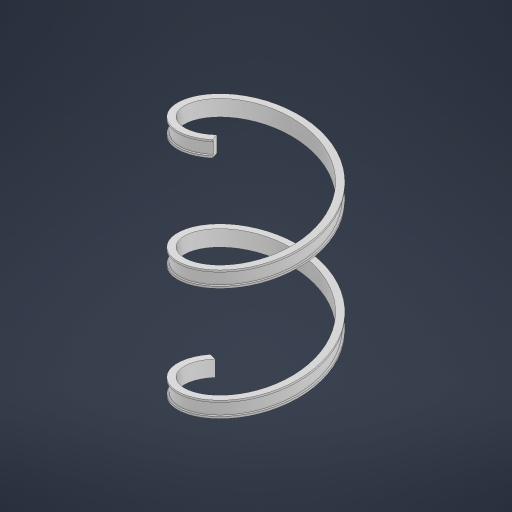
# Autodesk Inventor part: standalone
Saved by Autodesk Inventor 2023 (Build 270158000, 158)
## iProperties
Created: 2022-06-25
Part Number: standalone
Material: Generic
Document SubType Name: Modeling
Designer: bananenbrot
Density: 1 g/cm^3
Appearance: Default
Author: bananenbrot
Autodesk Inventor part; units mm, degrees
ref_plane "YZ Plane" through (0, 0, 0) normal (1, 0, 0) x (0, 1, 0)
ref_plane "XZ Plane" through (0, 0, 0) normal (0, 1, 0) x (-1, 0, 0)
ref_plane "XY Plane" through (0, 0, 0) normal (0, 0, 1) x (1, 0, 0)
sketch "Sketch1" plane through (0, 0, 0) normal (1, 0, 0) x (0, 1, 0)
  line L0 (-121.9366, 64.8131) -> (-121.9366, 71.8131)
  line L1 (-121.9366, 71.8131) -> (-119.9366, 71.8131)
  line L2 (-119.9366, 71.8131) -> (-119.9366, 69.8131)
  line L3 (-119.9366, 69.8131) -> (-106.9366, 69.8131)
  line L4 (-106.9366, 69.8131) -> (-106.9366, 71.8131)
  line L5 (-106.9366, 71.8131) -> (-104.9366, 71.8131)
  line L6 (-104.9366, 71.8131) -> (-104.9366, 64.8131)
  line L7 (-104.9366, 64.8131) -> (-121.9366, 64.8131)
  point P0 (0, 0)
  dimension "d7" = 13
  dimension "d8" = 2
  dimension "d9" = 2
  dimension "d10" = 2
  dimension "d11" = 5
  constraints: 16 end point, 6 perpendicular, 2 point on line
  measures "d7" distance of L2.end L3.end
  measures "d8" distance of L4.end L5.end
  measures "d9" distance of L0.end L1.end
  measures "d10" distance of L3.end L4.end
  measures "d11" distance between parallel lines of L7 L3
sketch3d "3D Sketch1"
  helix H0 starts at (19.0324, 12.1218, 67.3629) axis through (1.3595, 12.1218, 4.8116) along (0, -1, 0) pitch 120 turns 2.3333333 hand right
sweep "Sweep1" add profiles "Sketch1" path "3D Sketch1"
body "Solid1"
